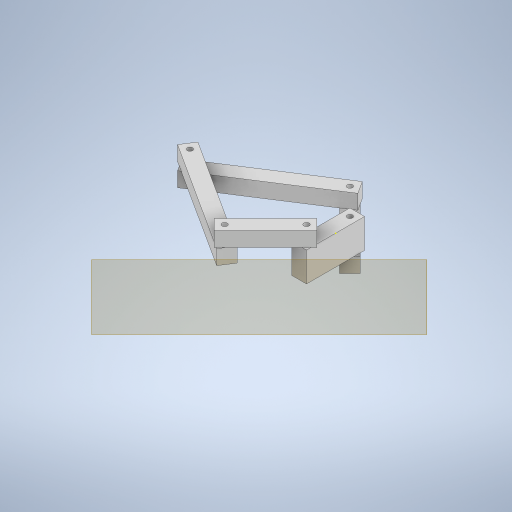
# Autodesk Inventor part: 5 Barras Simplificado
Saved by Autodesk Inventor 2024 (Build 280153000, 153)
## iProperties
Created: 2024-02-01
Part Number: 5 Barras Simplificado
Material: Generic
Document SubType Name: Modeling
Designer: juanp
Density: 1 g/cm^3
Appearance: Default
Author: juanp
Autodesk Inventor part; units mm, degrees
ref_plane "YZ Plane" through (0, 0, 0) normal (1, 0, 0) x (0, 1, 0)
ref_plane "XZ Plane" through (0, 0, 0) normal (0, 1, 0) x (-1, 0, 0)
ref_plane "XY Plane" through (0, 0, 0) normal (0, 0, 1) x (1, 0, 0)
sketch "Sketch1" plane through (0, 0, 0) normal (0, 1, 0) x (-1, 0, 0)
  line L0 (0, 75) -> (0, -75) construction
  line L1 (141.4214, 252.3424) -> (-35.921, 75)
  line L2 (-35.921, 75) -> (0, 39.079)
  line L3 (0, 39.079) -> (177.3424, 216.4214)
  line L4 (177.3424, 216.4214) -> (141.4214, 252.3424)
  circle A0 centre (141.4214, 216.4214) radius 25.4
  circle A1 centre (0, 75) radius 25.4
  circle A2 centre (141.4214, 216.4214) radius 9
  circle A3 centre (0, 75) radius 9
  line L5 (512.9205, 7.6183) -> (133.803, 251.5252)
  line L6 (133.803, 251.5252) -> (106.3175, 208.803)
  line L7 (106.3175, 208.803) -> (485.435, -35.1039)
  line L8 (485.435, -35.1039) -> (512.9205, 7.6183)
  circle A4 centre (477.8167, 0) radius 25.4
  circle A5 centre (141.4214, 216.4214) radius 25.4
  circle A6 centre (477.8167, 0) radius 9
  circle A7 centre (141.4214, 216.4214) radius 9
  line L9 (485.435, 35.1039) -> (106.3175, -208.803)
  line L10 (106.3175, -208.803) -> (133.803, -251.5252)
  line L11 (133.803, -251.5252) -> (512.9205, -7.6183)
  line L12 (512.9205, -7.6183) -> (485.435, 35.1039)
  circle A8 centre (477.8167, 0) radius 25.4
  circle A9 centre (141.4214, -216.4214) radius 25.4
  circle A10 centre (477.8167, 0) radius 9
  circle A11 centre (141.4214, -216.4214) radius 9
  line L13 (177.3424, -216.4214) -> (0, -39.079)
  line L14 (0, -39.079) -> (-35.921, -75)
  line L15 (-35.921, -75) -> (141.4214, -252.3424)
  line L16 (141.4214, -252.3424) -> (177.3424, -216.4214)
  circle A12 centre (141.4214, -216.4214) radius 25.4
  circle A13 centre (0, -75) radius 25.4
  circle A14 centre (141.4214, -216.4214) radius 9
  circle A15 centre (0, -75) radius 9
  circle A16 centre (0, -75) radius 25.4
  circle A17 centre (0, -75) radius 9
  line L17 (25.4, -100.4) -> (25.4, 100.4)
  line L18 (25.4, 100.4) -> (-25.4, 100.4)
  line L19 (-25.4, 100.4) -> (-25.4, -100.4)
  line L20 (-25.4, -100.4) -> (25.4, -100.4)
  circle A18 centre (0, -75) radius 25.4
  circle A19 centre (0, 75) radius 25.4
  circle A20 centre (0, -75) radius 9
  circle A21 centre (0, 75) radius 9
  line L21 (0, 75) -> (141.4214, 216.4214) construction
  line L22 (141.4214, 216.4214) -> (477.8167, 0) construction
  line L23 (477.8167, 0) -> (141.4214, -216.4214) construction
  line L24 (141.4214, -216.4214) -> (0, -75) construction
  line L25 (141.4214, 216.4214) -> (141.4214, 84) construction
  line L26 (309.619, -108.2107) -> (309.619, -234.619) construction
  line L27 (70.7107, -145.7107) -> (70.7107, -287.132)
  point P0 (0, 0)
  point P1 (0, 0)
  point P2 (70.7107, 145.7107)
  point P3 (309.619, 108.2107)
  dimension "d0" = 150
  dimension "d1" = 50.8
  dimension "d2" = 18
  dimension "d3" = 18
  dimension "d4" = 50.8
  dimension "d5" = 18
  dimension "d6" = 18
  dimension "d7" = 50.8
  dimension "d8" = 18
  dimension "d9" = 18
  dimension "d10" = 50.8
  dimension "d11" = 18
  dimension "d12" = 18
  dimension "d13" = 200
  dimension "d14" = 400
  dimension "d16" = 45
  dimension "d17" = 45
  dimension "d26" = 18
  dimension "d27" = 50.8
  dimension "d28" = 18
  dimension "d29" = 18
  dimension "d32" = 75
  dimension "d33" = 477.8166
  dimension "d34" = 145.7107
  dimension "d35" = 108.2107
  dimension "d36" = 70.7107
  dimension "d37" = 309.619
  dimension "d38" = 57.245
  dimension "d39" = 57.245
  dimension "d40" = 135
  constraints: 56 end point, 30 tangent, 22 centre point, 21 coincident, 10 parallel, 5 midpoint, 5 perpendicular, 4 vertical, 2 equal length
  measures "d0" distance of L0.start L0.end
  measures "d1" distance between parallel lines of L3 L1
  measures "d2" diameter of A2
  measures "d3" diameter of A3
  measures "d4" distance between parallel lines of L7 L5
  measures "d5" diameter of A6
  measures "d6" diameter of A7
  measures "d7" distance between parallel lines of L11 L9
  measures "d8" diameter of A10
  measures "d9" diameter of A11
  measures "d10" distance between parallel lines of L15 L13
  measures "d11" diameter of A14
  measures "d12" diameter of A15
  measures "d13" distance of A0.centre A1.centre
  measures "d14" distance of A4.centre A0.centre
  measures "d16" angle of L1 L0
  measures "d17" angle of L15 L0
  measures "d26" diameter of A17
  measures "d27" distance between parallel lines of L19 L17
  measures "d28" diameter of A20
  measures "d29" diameter of A21
  measures "d32" distance of point (0, 0) L0.start
  measures "d33" distance from line of L0 A4.centre
  measures "d34" vertical distance of point (70.711, 145.711) point (0, 0)
  measures "d35" vertical distance of point (309.619, 108.211) point (0, 0)
  measures "d36" horizontal distance of point (70.711, 145.711) point (0, 0)
  measures "d37" distance from line of point (309.619, 108.211) L0
  measures "d38" angle of L22 L25
  measures "d39" angle of L26 L23
  measures "d40" angle of L21 L0
extrude "Extrusion1" add sketch "Sketch1" along normal blind 50.8 contours L4 L5 L1 | L5 A0 L1 | L4 A0 L5 | A0 L6 L1 | A0 | L4 L3 A0 | L6 L7 L3 L17 L18 L1 | A0 L7 L6 | L18 A1 L1 | A0 L3 L7 | A1 L19 L1 | A1 | L18 L17 A1 | L19 L2 L1 | A1 L2 L19 | L17 L3 A1 | A1 L3 L2
extrude "Extrusion2" add sketch "Sketch1" against normal blind 50.8 separate body contours L5 A0 L1 | L1 L6 L5 | L5 L9 L7 L3 L4 | L4 A0 L5 | A0 L6 L1 | A0 | L4 L3 A0 | L5 A4 L9 | A0 L7 L6 | L5 L12 A4 | A4 | A4 L7 L9 | A0 L3 L7 | L5 L8 L12 | L12 L8 A4 | A4 L11 L7 | L11 L8 L7 | A4 L8 L11
sketch "Sketch2" plane through (0, -50.8, 0) normal (0, -1, 0) x (1, 0, 0)
  line L0 (35.921, 75) -> (0, 39.079) projected
  line L1 (35.921, 75) -> (0, 39.079) projected
  line L2 (0, 39.079) -> (-177.3424, 216.4214) projected
  line L3 (0, 39.079) -> (-177.3424, 216.4214) projected
  line L4 (-177.3424, 216.4214) -> (-141.4214, 252.3424) projected
  line L5 (-177.3424, 216.4214) -> (-141.4214, 252.3424) projected
  line L6 (-141.4214, 252.3424) -> (35.921, 75) projected
  line L7 (-141.4214, 252.3424) -> (35.921, 75) projected
  circle A0 centre (-141.4214, 216.4214) radius 9 projected
  circle A1 centre (-141.4214, 216.4214) radius 9 projected
  circle A2 centre (0, 75) radius 9 projected
  circle A3 centre (0, 75) radius 9 projected
  line L8 (35.921, 75) -> (0, 39.079) projected
  line L9 (-141.4214, 252.3424) -> (35.921, 75) projected
  line L10 (-177.3424, 216.4214) -> (-141.4214, 252.3424) projected
  line L11 (0, 39.079) -> (-177.3424, 216.4214) projected
  circle A4 centre (-141.4214, 216.4214) radius 9 projected
  circle A5 centre (0, 75) radius 9 projected
  line L12 (35.921, 75) -> (0, 39.079) projected
  line L13 (0, 39.079) -> (-177.3424, 216.4214) projected
  line L14 (-177.3424, 216.4214) -> (-141.4214, 252.3424) projected
  line L15 (-141.4214, 252.3424) -> (35.921, 75) projected
  circle A6 centre (-141.4214, 216.4214) radius 9 projected
  circle A7 centre (0, 75) radius 9 projected
  line L16 (35.921, 75) -> (0, 39.079) projected
  line L17 (35.921, 75) -> (0, 39.079) projected
  line L18 (0, 39.079) -> (-177.3424, 216.4214) projected
  line L19 (0, 39.079) -> (-177.3424, 216.4214) projected
  line L20 (-177.3424, 216.4214) -> (-141.4214, 252.3424) projected
  line L21 (-177.3424, 216.4214) -> (-141.4214, 252.3424) projected
  line L22 (-141.4214, 252.3424) -> (35.921, 75) projected
  line L23 (-141.4214, 252.3424) -> (35.921, 75) projected
  circle A8 centre (-141.4214, 216.4214) radius 9 projected
  circle A9 centre (-141.4214, 216.4214) radius 9 projected
  circle A10 centre (0, 75) radius 9 projected
  circle A11 centre (0, 75) radius 9 projected
  line L24 (-106.3175, 208.803) -> (-133.803, 251.5252) projected
  line L25 (-133.803, 251.5252) -> (-106.3175, 208.803) projected
  line L26 (-133.803, 251.5252) -> (-512.9205, 7.6183) projected
  line L27 (-512.9205, 7.6183) -> (-133.803, 251.5252) projected
  line L28 (-512.9205, 7.6183) -> (-485.435, -35.1039) projected
  line L29 (-485.435, -35.1039) -> (-512.9205, 7.6183) projected
  line L30 (-485.435, -35.1039) -> (-106.3175, 208.803) projected
  line L31 (-106.3175, 208.803) -> (-485.435, -35.1039) projected
  circle A12 centre (-477.8167, 0) radius 9 projected
  circle A13 centre (-477.8167, 0) radius 9 projected
  circle A14 centre (-141.4214, 216.4214) radius 9 projected
  circle A15 centre (-141.4214, 216.4214) radius 9 projected
  line L32 (-106.3175, 208.803) -> (-133.803, 251.5252) projected
  line L33 (-133.803, 251.5252) -> (-512.9205, 7.6183) projected
  line L34 (-512.9205, 7.6183) -> (-485.435, -35.1039) projected
  line L35 (-485.435, -35.1039) -> (-106.3175, 208.803) projected
  circle A16 centre (-477.8167, 0) radius 9 projected
  circle A17 centre (-141.4214, 216.4214) radius 9 projected
  line L36 (-133.803, 251.5252) -> (-106.3175, 208.803) projected
  line L37 (-106.3175, 208.803) -> (-485.435, -35.1039) projected
  line L38 (-485.435, -35.1039) -> (-512.9205, 7.6183) projected
  line L39 (-512.9205, 7.6183) -> (-133.803, 251.5252) projected
  circle A18 centre (-477.8167, 0) radius 9 projected
  circle A19 centre (-141.4214, 216.4214) radius 9 projected
  line L40 (-133.803, 251.5252) -> (-106.3175, 208.803) projected
  line L41 (-106.3175, 208.803) -> (-133.803, 251.5252) projected
  line L42 (-512.9205, 7.6183) -> (-133.803, 251.5252) projected
  line L43 (-133.803, 251.5252) -> (-512.9205, 7.6183) projected
  line L44 (-485.435, -35.1039) -> (-512.9205, 7.6183) projected
  line L45 (-512.9205, 7.6183) -> (-485.435, -35.1039) projected
  line L46 (-106.3175, 208.803) -> (-485.435, -35.1039) projected
  line L47 (-485.435, -35.1039) -> (-106.3175, 208.803) projected
  circle A20 centre (-477.8167, 0) radius 9 projected
  circle A21 centre (-477.8167, 0) radius 9 projected
  circle A22 centre (-141.4214, 216.4214) radius 9 projected
  circle A23 centre (-141.4214, 216.4214) radius 9 projected
  line L48 (0, -39.079) -> (35.921, -75) projected
  circle A24 centre (0, -75) radius 9 projected
  circle A25 centre (0, -75) radius 25.4 projected
  line L49 (35.921, -75) -> (-141.4214, -252.3424) projected
  line L50 (-177.3424, -216.4214) -> (0, -39.079) projected
  line L51 (-106.3175, -208.803) -> (-133.803, -251.5252) projected
  circle A26 centre (-141.4214, -216.4214) radius 9 projected
  circle A27 centre (-141.4214, -216.4214) radius 9 projected
  circle A28 centre (-141.4214, -216.4214) radius 25.4 projected
  circle A29 centre (-141.4214, -216.4214) radius 25.4 projected
  line L52 (-141.4214, -252.3424) -> (-177.3424, -216.4214) projected
  circle A30 centre (-477.8167, 0) radius 9 projected
  circle A31 centre (-477.8167, 0) radius 9 projected
  circle A32 centre (-477.8167, 0) radius 25.4 projected
  circle A33 centre (-477.8167, 0) radius 25.4 projected
  line L53 (0, 75) -> (0, -75) construction
  line L54 (35.921, 75) -> (0, 39.079) projected
  circle A34 centre (0, 75) radius 9 projected
  circle A35 centre (0, 75) radius 25.4 projected
  line L55 (0, 39.079) -> (-177.3424, 216.4214) projected
  line L56 (-141.4214, 252.3424) -> (35.921, 75) projected
  line L57 (-485.435, -35.1039) -> (-512.9205, 7.6183) projected
  line L58 (-512.9205, -7.6183) -> (-485.435, 35.1039) projected
  line L59 (-133.803, -251.5252) -> (-512.9205, -7.6183) projected
  line L60 (-485.435, 35.1039) -> (-106.3175, -208.803) projected
  circle A36 centre (-141.4214, 216.4214) radius 9 projected
  circle A37 centre (-141.4214, 216.4214) radius 9 projected
  line L61 (-177.3424, 216.4214) -> (-141.4214, 252.3424) projected
  line L62 (-106.3175, 208.803) -> (-485.435, -35.1039) projected
  line L63 (-512.9205, 7.6183) -> (-133.803, 251.5252) projected
  circle A38 centre (-141.4214, 216.4214) radius 25.4 projected
  circle A39 centre (-141.4214, 216.4214) radius 25.4 projected
  line L64 (-133.803, 251.5252) -> (-106.3175, 208.803) projected
  point P0 (0, 0)
  point P1 (0, 0)
  point P2 (0, 0)
  constraints: 9 other
extrude "Extrusion3" add sketch "Sketch2" along normal blind 50.8 separate body contours L60 L50 L52 L59 L30 | L30 A32 L60 | L30 L59 A32 | A32 | A32 L26 L60 | L60 A28 L50 | L59 L28 A32 | L26 L58 L60 | A32 L58 L26 | A28 L52 L50 | A28 | L60 L51 A28 | L52 A28 L59 | L28 L59 L58 | L28 L58 A32 | A28 L49 L59 | L51 L59 L49 | L49 A28 L51
sketch "Sketch3" plane through (0, -101.6, 0) normal (0, -1, 0) x (1, 0, 0)
  line L0 (35.921, 75) -> (0, 39.079) projected
  line L1 (35.921, 75) -> (0, 39.079) projected
  line L2 (0, 39.079) -> (-177.3424, 216.4214) projected
  line L3 (0, 39.079) -> (-177.3424, 216.4214) projected
  line L4 (-177.3424, 216.4214) -> (-141.4214, 252.3424) projected
  line L5 (-177.3424, 216.4214) -> (-141.4214, 252.3424) projected
  line L6 (-141.4214, 252.3424) -> (35.921, 75) projected
  line L7 (-141.4214, 252.3424) -> (35.921, 75) projected
  circle A0 centre (-141.4214, 216.4214) radius 9 projected
  circle A1 centre (-141.4214, 216.4214) radius 9 projected
  circle A2 centre (0, 75) radius 9 projected
  circle A3 centre (0, 75) radius 9 projected
  line L8 (35.921, 75) -> (0, 39.079) projected
  line L9 (-141.4214, 252.3424) -> (35.921, 75) projected
  line L10 (-177.3424, 216.4214) -> (-141.4214, 252.3424) projected
  line L11 (0, 39.079) -> (-177.3424, 216.4214) projected
  circle A4 centre (-141.4214, 216.4214) radius 9 projected
  circle A5 centre (0, 75) radius 9 projected
  line L12 (35.921, 75) -> (0, 39.079) projected
  line L13 (0, 39.079) -> (-177.3424, 216.4214) projected
  line L14 (-177.3424, 216.4214) -> (-141.4214, 252.3424) projected
  line L15 (-141.4214, 252.3424) -> (35.921, 75) projected
  circle A6 centre (-141.4214, 216.4214) radius 9 projected
  circle A7 centre (0, 75) radius 9 projected
  line L16 (35.921, 75) -> (0, 39.079) projected
  line L17 (35.921, 75) -> (0, 39.079) projected
  line L18 (0, 39.079) -> (-177.3424, 216.4214) projected
  line L19 (0, 39.079) -> (-177.3424, 216.4214) projected
  line L20 (-177.3424, 216.4214) -> (-141.4214, 252.3424) projected
  line L21 (-177.3424, 216.4214) -> (-141.4214, 252.3424) projected
  line L22 (-141.4214, 252.3424) -> (35.921, 75) projected
  line L23 (-141.4214, 252.3424) -> (35.921, 75) projected
  circle A8 centre (-141.4214, 216.4214) radius 9 projected
  circle A9 centre (-141.4214, 216.4214) radius 9 projected
  circle A10 centre (0, 75) radius 9 projected
  circle A11 centre (0, 75) radius 9 projected
  line L24 (-106.3175, 208.803) -> (-133.803, 251.5252) projected
  line L25 (-133.803, 251.5252) -> (-106.3175, 208.803) projected
  line L26 (-133.803, 251.5252) -> (-512.9205, 7.6183) projected
  line L27 (-512.9205, 7.6183) -> (-133.803, 251.5252) projected
  line L28 (-512.9205, 7.6183) -> (-485.435, -35.1039) projected
  line L29 (-485.435, -35.1039) -> (-512.9205, 7.6183) projected
  line L30 (-485.435, -35.1039) -> (-106.3175, 208.803) projected
  line L31 (-106.3175, 208.803) -> (-485.435, -35.1039) projected
  circle A12 centre (-477.8167, 0) radius 9 projected
  circle A13 centre (-477.8167, 0) radius 9 projected
  circle A14 centre (-141.4214, 216.4214) radius 9 projected
  circle A15 centre (-141.4214, 216.4214) radius 9 projected
  line L32 (-106.3175, 208.803) -> (-133.803, 251.5252) projected
  line L33 (-133.803, 251.5252) -> (-512.9205, 7.6183) projected
  line L34 (-512.9205, 7.6183) -> (-485.435, -35.1039) projected
  line L35 (-485.435, -35.1039) -> (-106.3175, 208.803) projected
  circle A16 centre (-477.8167, 0) radius 9 projected
  circle A17 centre (-141.4214, 216.4214) radius 9 projected
  line L36 (-133.803, 251.5252) -> (-106.3175, 208.803) projected
  line L37 (-106.3175, 208.803) -> (-485.435, -35.1039) projected
  line L38 (-485.435, -35.1039) -> (-512.9205, 7.6183) projected
  line L39 (-512.9205, 7.6183) -> (-133.803, 251.5252) projected
  circle A18 centre (-477.8167, 0) radius 9 projected
  circle A19 centre (-141.4214, 216.4214) radius 9 projected
  line L40 (-133.803, 251.5252) -> (-106.3175, 208.803) projected
  line L41 (-106.3175, 208.803) -> (-133.803, 251.5252) projected
  line L42 (-512.9205, 7.6183) -> (-133.803, 251.5252) projected
  line L43 (-133.803, 251.5252) -> (-512.9205, 7.6183) projected
  line L44 (-485.435, -35.1039) -> (-512.9205, 7.6183) projected
  line L45 (-512.9205, 7.6183) -> (-485.435, -35.1039) projected
  line L46 (-106.3175, 208.803) -> (-485.435, -35.1039) projected
  line L47 (-485.435, -35.1039) -> (-106.3175, 208.803) projected
  circle A20 centre (-477.8167, 0) radius 9 projected
  circle A21 centre (-477.8167, 0) radius 9 projected
  circle A22 centre (-141.4214, 216.4214) radius 9 projected
  circle A23 centre (-141.4214, 216.4214) radius 9 projected
  line L48 (-512.9205, -7.6183) -> (-133.803, -251.5252) projected
  line L49 (-512.9205, -7.6183) -> (-133.803, -251.5252) projected
  line L50 (-133.803, -251.5252) -> (-106.3175, -208.803) projected
  line L51 (-133.803, -251.5252) -> (-106.3175, -208.803) projected
  line L52 (-106.3175, -208.803) -> (-485.435, 35.1039) projected
  line L53 (-106.3175, -208.803) -> (-485.435, 35.1039) projected
  line L54 (-485.435, 35.1039) -> (-512.9205, -7.6183) projected
  line L55 (-485.435, 35.1039) -> (-512.9205, -7.6183) projected
  circle A24 centre (-141.4214, -216.4214) radius 9 projected
  circle A25 centre (-141.4214, -216.4214) radius 9 projected
  circle A26 centre (-477.8167, 0) radius 9 projected
  circle A27 centre (-477.8167, 0) radius 9 projected
  line L56 (-512.9205, -7.6183) -> (-133.803, -251.5252) projected
  line L57 (-485.435, 35.1039) -> (-512.9205, -7.6183) projected
  line L58 (-106.3175, -208.803) -> (-485.435, 35.1039) projected
  line L59 (-133.803, -251.5252) -> (-106.3175, -208.803) projected
  circle A28 centre (-141.4214, -216.4214) radius 9 projected
  circle A29 centre (-477.8167, 0) radius 9 projected
  line L60 (-512.9205, -7.6183) -> (-133.803, -251.5252) projected
  line L61 (-133.803, -251.5252) -> (-106.3175, -208.803) projected
  line L62 (-106.3175, -208.803) -> (-485.435, 35.1039) projected
  line L63 (-485.435, 35.1039) -> (-512.9205, -7.6183) projected
  circle A30 centre (-141.4214, -216.4214) radius 9 projected
  circle A31 centre (-477.8167, 0) radius 9 projected
  line L64 (-512.9205, -7.6183) -> (-133.803, -251.5252) projected
  line L65 (-512.9205, -7.6183) -> (-133.803, -251.5252) projected
  line L66 (-133.803, -251.5252) -> (-106.3175, -208.803) projected
  line L67 (-133.803, -251.5252) -> (-106.3175, -208.803) projected
  line L68 (-106.3175, -208.803) -> (-485.435, 35.1039) projected
  line L69 (-106.3175, -208.803) -> (-485.435, 35.1039) projected
  line L70 (-485.435, 35.1039) -> (-512.9205, -7.6183) projected
  line L71 (-485.435, 35.1039) -> (-512.9205, -7.6183) projected
  circle A32 centre (-141.4214, -216.4214) radius 9 projected
  circle A33 centre (-141.4214, -216.4214) radius 9 projected
  circle A34 centre (-477.8167, 0) radius 9 projected
  circle A35 centre (-477.8167, 0) radius 9 projected
  line L72 (0, -39.079) -> (35.921, -75) projected
  circle A36 centre (0, -75) radius 9 projected
  circle A37 centre (0, -75) radius 25.4 projected
  line L73 (35.921, -75) -> (-141.4214, -252.3424) projected
  line L74 (-177.3424, -216.4214) -> (0, -39.079) projected
  line L75 (-106.3175, -208.803) -> (-133.803, -251.5252) projected
  circle A38 centre (-141.4214, -216.4214) radius 9 projected
  circle A39 centre (-141.4214, -216.4214) radius 9 projected
  circle A40 centre (-141.4214, -216.4214) radius 25.4 projected
  circle A41 centre (-141.4214, -216.4214) radius 25.4 projected
  line L76 (-141.4214, -252.3424) -> (-177.3424, -216.4214) projected
  circle A42 centre (-477.8167, 0) radius 9 projected
  circle A43 centre (-477.8167, 0) radius 9 projected
  circle A44 centre (-477.8167, 0) radius 25.4 projected
  circle A45 centre (-477.8167, 0) radius 25.4 projected
  line L77 (0, 75) -> (0, -75) construction
  line L78 (35.921, 75) -> (0, 39.079) projected
  circle A46 centre (0, 75) radius 9 projected
  circle A47 centre (0, 75) radius 25.4 projected
  line L79 (0, 39.079) -> (-177.3424, 216.4214) projected
  line L80 (-141.4214, 252.3424) -> (35.921, 75) projected
  line L81 (-485.435, -35.1039) -> (-512.9205, 7.6183) projected
  line L82 (-512.9205, -7.6183) -> (-485.435, 35.1039) projected
  line L83 (-133.803, -251.5252) -> (-512.9205, -7.6183) projected
  line L84 (-485.435, 35.1039) -> (-106.3175, -208.803) projected
  circle A48 centre (-141.4214, 216.4214) radius 9 projected
  circle A49 centre (-141.4214, 216.4214) radius 9 projected
  line L85 (-177.3424, 216.4214) -> (-141.4214, 252.3424) projected
  line L86 (-106.3175, 208.803) -> (-485.435, -35.1039) projected
  line L87 (-512.9205, 7.6183) -> (-133.803, 251.5252) projected
  circle A50 centre (-141.4214, 216.4214) radius 25.4 projected
  circle A51 centre (-141.4214, 216.4214) radius 25.4 projected
  line L88 (-133.803, 251.5252) -> (-106.3175, 208.803) projected
  point P0 (0, 0)
  point P1 (0, 0)
  point P2 (0, 0)
  constraints: 13 other
extrude "Extrusion4" add sketch "Sketch3" along normal blind 50.8 separate body contours L74 A37 L73 L50 L52 | L52 A40 L74 | L52 L50 A40 | A40 | A40 L76 L74 | L74 L72 A37 | A37 | L76 A40 L48 | L48 L73 L76 | L72 L73 A37 | A40 L73 L48 | L50 L73 A40
extrude "Extrusion5" add sketch "Sketch1" against normal blind 101.6 separate body contours L18 A1 L1 | L1 L19 L18 | A1 L19 L1 | A1 | L18 L17 A1 | A1 L2 L19 | L17 L3 A1 | L17 L13 L14 L19 L2 L3 | L17 A13 L13 | A1 L3 L2 | A13 L14 L13 | A13 | L17 L20 A13 | L14 A13 L19 | L20 L15 A13 | A13 L15 L19 | L15 L20 L19
sketch "Sketch4" plane through (25.4, 0, 100.4) normal (1, 0, 0) x (0, 0, -1)
  point P0 (100.4, 0)
ref_plane "Work Plane1" through (133.5018, 0, 172.5807) normal (0.7071068, 0, 0.7071068) x (0.7071068, 0, -0.7071068)
body "Solid1"
body "Solid2"
body "Solid3"
body "Solid4"
body "Solid5"
